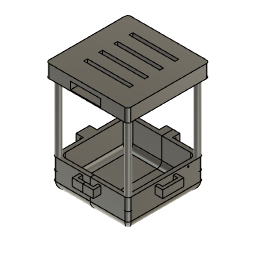
hydro3k-v1.0 v16 (Autodesk Fusion 360 design; units mm, degrees)
Autodesk Fusion 360 part; units mm, degrees
sketch "Bottom" plane through (0, 0, 0) normal (0, 0, 1) x (1, 0, 0)
  line L0 (0, 0) -> (250, 0)
  line L1 (250, 0) -> (250, 250)
  line L2 (250, 250) -> (0, 250)
  line L3 (0, 250) -> (0, 0)
  dimension "d1" = 250
  dimension "d2" = 250
  constraint horizontal L0
  constraint vertical L1
  constraint horizontal L2
  constraint vertical L3
  constraint coincident L0.start L3.end
  measures "d1" distance of L0.end L1.end
  measures "d2" distance of L1.end L2.end
extrude "Extrude1" add sketch "Bottom" along normal blind 60 makes body 1
shell "Shell1" thickness 13 removed faces 1 at (83.3333, 166.6667, 60) on bodies 1
fillet "Fillet1" radius 16 2 edges at (125, 237, 13) (13, 125, 13) on bodies 1
fillet "Fillet2" radius 16 3 edges at (237, 117, 13) (237, 232.3137, 17.6863) (237, 237, 44.5) on bodies 1
fillet "Fillet3" radius 16 2 edges at (17.6863, 232.3137, 17.6863) (13, 237, 44.5) on bodies 1
fillet "Fillet4" radius 16 5 edges at (237, 13, 44.5) (232.3137, 13, 17.6863) (125, 13, 13) (17.6863, 13, 17.6863) (13, 13, 44.5) on bodies 1
fillet "Fillet5" radius 10 4 edges at (250, 250, 30) (0, 250, 30) (250, 0, 30) (0, 0, 30) on bodies 1
fillet "Fillet6" radius 30 8 edges at (247.0711, 247.0711, 0) (125, 250, 0) (2.9289, 247.0711, 0) (0, 125, 0) (2.9289, 2.9289, 0) (125, 0, 0) (247.0711, 2.9289, 0) (250, 125, 0) on bodies 1
sketch "Pillar" plane through (0, 0, 60) normal (0, 0, 1) x (-1, 0, 0)
  arc A0 (0, -10) -> (-10, 0) centre (-10, -10) ccw
  line L0 (-10, 0) -> (-240, 0)
  arc A1 (-240, 0) -> (-250, -10) centre (-240, -10) ccw
  line L1 (-250, -10) -> (-250, -240)
  arc A2 (-250, -240) -> (-240, -250) centre (-240, -240) ccw
  line L2 (-240, -250) -> (-10, -250)
  arc A3 (-10, -250) -> (0, -240) centre (-10, -240) ccw
  line L3 (0, -240) -> (0, -10)
  line L4 (-29, -237) -> (-221, -237)
  arc A4 (-237, -221) -> (-221, -237) centre (-221, -221) ccw
  line L5 (-237, -221) -> (-237, -29)
  arc A5 (-221, -13) -> (-237, -29) centre (-221, -29) ccw
  line L6 (-221, -13) -> (-29, -13)
  arc A6 (-13, -29) -> (-29, -13) centre (-29, -29) ccw
  line L7 (-13, -29) -> (-13, -221)
  arc A7 (-29, -237) -> (-13, -221) centre (-29, -221) ccw
  circle A8 through (-0.0675, -9.6691, 5) (-14.5058, -1.3332, 5) (-14.5058, -18.0051, 5)
  dimension "d18" = 19.2511
extrude "Extrude2" add sketch "Pillar" along normal blind 300 separate body contours A8 in plane through (0, 0, 65) normal (0, 0, 1) makes body 2
copy_body "CopyPasteBodies1" bodies 2 makes body 3
move_body "Move1" bodies 3 to x (1, 0, 0) y (0, 1, 0) z (0, 0, 1) at (230.7, 0, -5)
copy_body "CopyPasteBodies2" bodies 3 makes body 4
move_body "Move2" bodies 4 to x (1, 0, 0) y (0, 1, 0) z (0, 0, 1) at (-0.2, 230.7, 0)
move_body "Move3" bodies 2 to x (1, 0, 0) y (0, 1, 0) z (0, 0, 1) at (0, 0.0299, -5)
copy_body "CopyPasteBodies3" bodies 2 makes body 5
move_body "Move4" bodies 5 to x (1, 0, 0) y (0, 1, 0) z (0, 0, 1) at (0.0538, 230.5628, 0)
move_body "Move5" bodies 2 to x (1, 0, 0) y (0, 1, 0) z (0, 0, 1) at (0.0788, 0.0315, 0)
extrude "Extrude3" add sketch "Bottom" along normal blind 40 separate body makes body 6
move_body "Move6" bodies 6 to x (1, 0, 0) y (0, 1, 0) z (0, 0, 1) at (0, 0, 325)
fillet "Fillet7" radius 9 2 edges at (250, 250, 345) (0, 250, 345) on bodies 6
fillet "Fillet8" radius 9 2 edges at (0, 0, 345) (250, 0, 345) on bodies 6
scale "Scale1" factor 1.08444 about (250, 9, 325) bodies 6
move_body "Move7" bodies 6 to x (1, 0, 0) y (0, 1, 0) z (0, 0, 1) at (10, -10, 0)
copy_body "CopyPasteBodies4" bodies 5 makes body 7
move_body "Move8" bodies 7 to x (1, 0, 0) y (0, 1, 0) z (0, 0, 1) at (0, -20, 0)
move_body "Move9" bodies 7 to x (1, 0, 0) y (0, 1, 0) z (0, 0, 1) at (0, 20, 0)
extrude "Extrude7" cut 1 faces at (4.6943, 240.6827, 360) along direction (0, 0, -1) blind 40 on bodies 7 bodies 7
extrude "Extrude8" cut 1 faces at (4.6943, 240.6827, 320) along direction (0, 0, 1) blind 40 on bodies 7 bodies 6
delete_body "RemoveBody1" bodies 7
combine "Combine1" operation cut target body 6 tool bodies 2 keep tools
combine "Combine2" operation cut target body 6 tool bodies 3 4 keep tools
fillet "Fillet10" radius 5 1 edges at (18.721, 243.7426, 360) 4 faces at (8.7844, 7.9691, 360) (245.678, 11.1645, 360) (237.5842, 240.8473, 360) (4.6943, 240.6827, 360) on bodies 2 3 4 5
sketch "Top punch" plane through (0, 0, 368.3776) normal (0, 0, 1) x (-1, 0, 0)
  arc A0 (-250.24, 10.76) -> (-260, 1) centre (-250.24, 1) ccw
  line L0 (-260, 1) -> (-260, -250.5901)
  arc A1 (-260, -250.5901) -> (-250.24, -260.35) centre (-250.24, -250.5901) ccw
  line L1 (-250.24, -260.35) -> (1.35, -260.35)
  arc A2 (1.35, -260.35) -> (11.11, -250.5901) centre (1.35, -250.5901) ccw
  line L2 (11.11, -250.5901) -> (11.11, 1)
  arc A3 (11.11, 1) -> (1.35, 10.76) centre (1.35, 1) ccw
  line L3 (1.35, 10.76) -> (-250.24, 10.76)
  line L4 (-201.4485, -54.1081) -> (-49.4485, -54.1081)
  line L5 (-49.4485, -54.1081) -> (-49.4485, -66.1081)
  line L6 (-49.4485, -66.1081) -> (-201.4485, -66.1081)
  line L7 (-201.4485, -66.1081) -> (-201.4485, -54.1081)
  line L8 (-201.4485, -104.1081) -> (-49.4485, -104.1081)
  line L9 (-201.4485, -116.1081) -> (-201.4485, -104.1081)
  line L10 (-49.4485, -116.1081) -> (-201.4485, -116.1081)
  line L11 (-49.4485, -104.1081) -> (-49.4485, -116.1081)
  line L12 (-201.4485, -154.1081) -> (-49.4485, -154.1081)
  line L13 (-201.4485, -166.1081) -> (-201.4485, -154.1081)
  line L14 (-49.4485, -166.1081) -> (-201.4485, -166.1081)
  line L15 (-49.4485, -154.1081) -> (-49.4485, -166.1081)
  line L16 (-201.4485, -204.1081) -> (-49.4485, -204.1081)
  line L17 (-201.4485, -216.1081) -> (-201.4485, -204.1081)
  line L18 (-49.4485, -216.1081) -> (-201.4485, -216.1081)
  line L19 (-49.4485, -204.1081) -> (-49.4485, -216.1081)
  dimension "d46" = 0
  dimension "d47" = -150
  constraint horizontal L4
  constraint vertical L5
  constraint horizontal L6
  constraint vertical L7
extrude "Extrude10" cut sketch "Top punch" against normal blind 15 contours L4 L5 L6 L7 | L8 L9 L10 L11 | L12 L13 L14 L15 | L16 L17 L18 L19 bodies 6
move_body "Move10" bodies 1 5 3 2 4 6 to x (1, 0, 0) y (0, 1, 0) z (0, 0, 1) at (0, 0, 368)
extrude "Extrude11" add sketch "Top punch" against normal blind 11 contours L4 L5 L6 L7 | L8 L9 L10 L11 | L12 L13 L14 L15 | L16 L17 L18 L19 bodies 1
move_body "Move11" bodies 5 6 4 2 3 1 to x (1, 0, 0) y (0, 1, 0) z (0, 0, 1) at (0, 0, -356)
extrude "Extrude12" add 1 faces at (4.3333, 157, 72) along direction (0, 0, 1) blind 40 on bodies 1 bodies 1
sketch "Sketch5" plane through (250, 0, 0) normal (1, 0, 0) x (0, 1, 0)
  line L0 (10, 42) -> (240, 42)
  line L1 (240, 42) -> (240, 112)
  line L2 (240, 112) -> (10, 112)
  line L3 (10, 112) -> (10, 42)
  circle A0 centre (200, 105) radius 2.5
  dimension "d67" = 5
  measures "d67" diameter of A0
hole "Hole1" at (250, 200, 105) direction (-1, 0, 0) diameter 5 depth 40 tip angle 18 bodies 1
sketch "Sketch6" plane through (0, 0, 0) normal (0, 0, 1) x (1, 0, 0)
  line L0 (0, 25) -> (0, 0)
  line L1 (0, 0) -> (70, 0)
  line L2 (70, 0) -> (70, 25)
  line L3 (70, 25) -> (60, 25)
  line L4 (60, 25) -> (60, 10)
  line L5 (60, 10) -> (10, 10)
  line L6 (10, 10) -> (10, 25)
  line L7 (10, 25) -> (0, 25)
  constraint coincident L0.end L1.start
  constraint vertical L0
  constraint perpendicular L0 L1
  constraint perpendicular L1 L2
  constraint perpendicular L0 L3
  constraint perpendicular L3 L4
  constraint perpendicular L4 L5
  constraint perpendicular L5 L6
extrude "Extrude13" add sketch "Sketch6" along normal blind 25 separate body makes body 8
move_body "Move12" bodies 8 to x (1, 0, 0) y (0, 1, 0) z (0, 0, 1) at (90, -25, 80)
copy_body "CopyPasteBodies5" bodies 8 makes body 9
move_body "Move13" bodies 9 to x (1, 0, 0) y (0, 1, 0) z (0, 0, 1) at (150, 120, 0)
move_body "Move14" bodies 9 to x (0, 1, 0) y (-1, 0, 0) z (0, 0, 1) at (370, -130, 0)
move_body "Move15" bodies 9 to x (1, 0, 0) y (0, 1, 0) z (0, 0, 1) at (0, -20, 0)
sketch "Sketch7" plane through (0, 0, 0) normal (1, 0, 0) x (0, 1, 0)
  line L0 (0, 31) -> (11, 31)
  line L1 (11, 31) -> (24, 31)
  line L2 (24, 31) -> (24, 0)
  line L3 (24, 0) -> (11, 0)
  line L4 (11, 0) -> (11, 25)
  line L5 (11, 25) -> (0, 25)
  line L6 (0, 25) -> (0, 31)
  dimension "d77" = 13
  constraint horizontal L0
  constraint parallel L0 L1
  constraint perpendicular L1 L2
  constraint perpendicular L2 L3
  constraint perpendicular L3 L4
  constraint perpendicular L4 L5
  constraint perpendicular L0 L6
  measures "d77" distance of L0.end L1.end
extrude "Extrude14" add sketch "Sketch7" along normal blind 45 separate body makes body 10
move_body "Move16" bodies 10 to x (1, 0, 0) y (0, 1, 0) z (0, 0, 1) at (103, -25, 70)
move_body "Move17" bodies 10 to x (1, 0, 0) y (0, 1, 0) z (0, 0, 1) at (0, 0, 11)
move_body "Move18" bodies 10 to x (1, 0, 0) y (0, 1, 0) z (0, 0, 1) at (0, 275, 0)
copy_body "CopyPasteBodies6" bodies 10 makes body 11
move_body "Move19" bodies 11 to x (0, 1, 0) y (-1, 0, 0) z (0, 0, 1) at (353, 147, 0)
move_body "Move20" bodies 11 to x (1, 0, 0) y (0, 1, 0) z (0, 0, 1) at (-103, -148, 0)
sketch "Sketch8" plane through (0, -10.76, 0) normal (0, -1, 0) x (1, 0, 0)
  line L0 (250.24, 337) -> (250.24, 380.3776)
  line L1 (250.24, 380.3776) -> (-1.35, 380.3776)
  line L2 (-1.35, 380.3776) -> (-1.35, 337)
  line L3 (-1.35, 337) -> (250.24, 337)
  line L4 (70, 365) -> (70, 340)
  line L5 (70, 340) -> (170, 340)
  line L6 (170, 340) -> (170, 365)
  line L7 (170, 365) -> (70, 365)
  constraint perpendicular L1 L4
  constraint perpendicular L4 L5
  constraint perpendicular L1 L6
  constraint perpendicular L4 L7
extrude "Extrude15" cut sketch "Sketch8" against normal blind 80 contours L4 L5 L6 L7 bodies 6
combine "Combine3" operation add target body 1 tool bodies 9 11 10
combine "Combine4" operation add target body 8 tool bodies 1
copy_body "Body->Comp1" bodies 2 removing the originals makes body 12 in component "pillar-1"
copy_body "Body->Comp2" bodies 4 removing the originals makes body 13 in component "pillar-3"
copy_body "Body->Comp3" bodies 5 removing the originals makes body 14 in component "pillar-4"
copy_body "Body->Comp4" bodies 3 removing the originals makes body 15 in component "pillar-2"
copy_body "Body->Comp5" bodies 8 removing the originals makes body 16 in component "res"
sketch "Sketch10" plane through (0, 0, 0) normal (0, 0, 1) x (1, 0, 0)
  line L0 (148, 250) -> (148, 274)
  line L1 (148, 274) -> (127, 274)
  line L2 (127, 274) -> (127, 248.619)
  line L3 (127, 248.619) -> (143.3302, 248.619)
  line L4 (143.3302, 248.619) -> (143.3302, 223.619)
  line L5 (143.3302, 223.619) -> (126.7415, 223.619)
  line L6 (126.7415, 223.619) -> (126.7415, 198.619)
  line L7 (126.7415, 198.619) -> (151.268, 198.619)
  line L8 (151.268, 198.619) -> (151.268, 173.619)
  line L9 (151.268, 173.619) -> (126.7415, 173.619)
  line L10 (126.7415, 173.619) -> (126.7415, 148.619)
  line L11 (126.7415, 148.619) -> (151.268, 148.619)
  line L12 (151.268, 148.619) -> (151.268, 123.619)
  line L13 (151.268, 123.619) -> (126.7415, 123.619)
  line L14 (126.7415, 123.619) -> (126.7415, 98.619)
  line L15 (126.7415, 98.619) -> (151.268, 98.619)
  line L16 (151.268, 98.619) -> (151.268, 73.619)
  line L17 (151.268, 73.619) -> (126.7415, 73.619)
  line L18 (126.7415, 73.619) -> (126.7415, 48.619)
  line L19 (126.7415, 48.619) -> (151.268, 48.619)
  line L20 (151.268, 48.619) -> (151.268, 23.619)
  line L21 (151.268, 23.619) -> (126.7415, 23.619)
  line L22 (150, -15) -> (126.8725, -15)
  line L23 (126.8725, -15) -> (126.8725, -20.9133)
  line L24 (126.8725, -20.9133) -> (157.1675, -20.9133)
  line L25 (157.1675, -20.9133) -> (157.1675, 250)
  line L26 (157.1675, 250) -> (148, 250)
  line L27 (150, -15) -> (150, 0)
  line L28 (150, 0) -> (126.8725, 0)
  line L29 (126.8725, 0) -> (126.7415, 23.619)
  constraint vertical L0
  constraint perpendicular L0 L1
  constraint perpendicular L1 L2
  constraint perpendicular L0 L3
  constraint perpendicular L3 L4
  constraint perpendicular L4 L5
  constraint perpendicular L5 L6
  constraint perpendicular L6 L7
  constraint perpendicular L7 L8
  constraint perpendicular L8 L9
  constraint perpendicular L9 L10
  constraint perpendicular L10 L11
  constraint perpendicular L11 L12
  constraint perpendicular L12 L13
  constraint perpendicular L13 L14
  constraint perpendicular L14 L15
  constraint perpendicular L15 L16
  constraint perpendicular L16 L17
  constraint perpendicular L17 L18
  constraint perpendicular L18 L19
  constraint perpendicular L19 L20
  constraint perpendicular L20 L21
  constraint perpendicular L22 L23
  constraint perpendicular L23 L24
  constraint perpendicular L24 L25
  constraint horizontal L22
  constraint perpendicular L22 L27
  constraint perpendicular L23 L28
ref_plane "WorkPlane4" through (125, 125, 77) normal (-1, 0, 0) x (0, -1, 0)
split "Split1" by plane through (125, 125, 77) normal (-1, 0, 0) bodies 16 makes body 17 at (61, 93, 25) in component "res"
sketch "Sketch9" plane through (0, 0, 0) normal (0, 0, 1) x (1, 0, 0)
component "pillar-1" placed x (1, 0, 0) y (0, 1, 0) z (0, 0, 1) at (0, 0, 0)
component "pillar-3" placed x (1, 0, 0) y (0, 1, 0) z (0, 0, 1) at (0, 0, 0)
component "pillar-4" placed x (1, 0, 0) y (0, 1, 0) z (0, 0, 1) at (0, 0, 0)
component "pillar-2" placed x (1, 0, 0) y (0, 1, 0) z (0, 0, 1) at (0, 0, 0)
component "res" placed x (1, 0, 0) y (0, 1, 0) z (0, 0, 1) at (0, 0, 0)
named bodies: "pillar", "pillar (1)", "pillar-1", "topp", "pillar-1 (1)", "pillar-1 (1) (1)", "res", "handle", "pillar-3", "pillar-4", "pillar-2", "res (1)"
